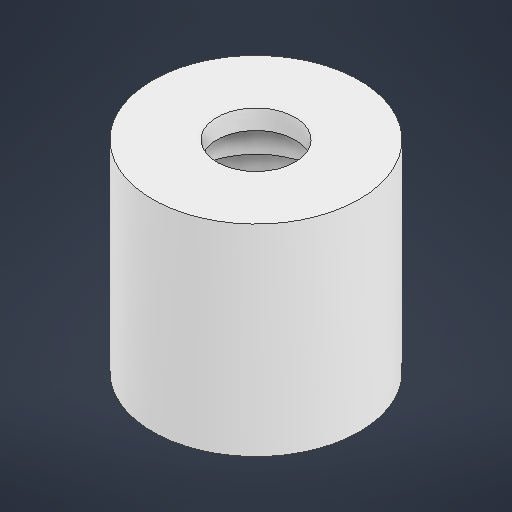
# Autodesk Inventor part: limite
Saved by Autodesk Inventor 2026.1 (Build 301233020, 233B)
## iProperties
Created: 2025-10-22
Part Number: limite
Material: Plástico ABS
Document SubType Name: Modeling
Designer: rodri
Density: 1.06 g/cm^3
Appearance: Suave - Blanco
Author: rodri
## iProperties of the stored document limite_3DPrint.ipt
Created: 2025-10-22
Part Number: limite_3DPrint
Material: Genérico
Document SubType Name: Modeling
Designer: rodri
Density: 1 g/cm^3
Appearance: Valor por defecto
Author: rodri
Autodesk Inventor part; units mm, degrees
ref_plane "YZ Plane" through (0, 0, 0) normal (1, 0, 0) x (0, 1, 0)
ref_plane "XZ Plane" through (0, 0, 0) normal (0, 1, 0) x (-1, 0, 0)
ref_plane "XY Plane" through (0, 0, 0) normal (0, 0, 1) x (1, 0, 0)
sketch "Boceto1" plane through (0, 0, 0) normal (0, 1, 0) x (-1, 0, 0)
  circle A0 centre (0, 0) radius 14.4
  circle A1 centre (0, 0) radius 15.9
  dimension "d0" = 28.8
  dimension "d1" = 1.5
  constraints: 2 centre point, 1 coincident
  measures "d0" diameter of A0
  measures "d1" radial gap between concentric circles of A0 A1
extrude "Extrusión1" add sketch "Boceto1" along normal blind 22
sketch "Boceto2" plane through (0, 0, 0) normal (0, 0, 1) x (1, 0, 0)
  line L0 (15.9, 22) -> (-15.9, 22) projected
  point P0 (0, 0)
  point P1 (0, 7)
  dimension "d4" = 15
  measures "d4" distance from line of point (0, 7) L0
hole "Agujero1" at (0, 7, 0) direction (0, 0, -1) diameter 7 end through all clearance for "Tornillo para maquinaria de cabeza plana" size "M6" standard "Perfil M métrico ANSI"
sketch "Boceto3" plane through (0, 22, 0) normal (0, 1, 0) x (1, 0, 0)
  circle A0 centre (0, 0) radius 15.9 projected
  circle A1 centre (0, 0) radius 10
  dimension "d12" = 20
  constraints: 1 centre point, 1 coincident
  measures "d12" diameter of A1
extrude "Extrusión2" add sketch "Boceto3" along normal blind 6
sketch "Boceto4" plane through (0, 28, 0) normal (0, 1, 0) x (1, 0, 0)
  circle A0 centre (0, 0) radius 15.9 projected
  circle A1 centre (0, 0) radius 6
  dimension "d15" = 12
  constraints: 1 centre point, 1 coincident
  measures "d15" diameter of A1
extrude "Extrusión3" add sketch "Boceto4" along normal blind 3
